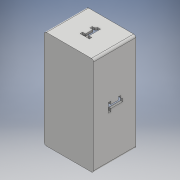
# Autodesk Inventor part: Контейнер 1
Saved by Autodesk Inventor 2018 (Build 220112000, 112)
## iProperties
Created: 2023-02-08
Part Number: Контейнер 1
Material: Типовые
Document SubType Name: Modeling
Designer: exper
Density: 1 g/cm^3
Appearance: По умолчанию
Author: exper
Autodesk Inventor part; units mm, degrees
ref_plane "YZ Plane" through (0, 0, 0) normal (1, 0, 0) x (0, 1, 0)
ref_plane "XZ Plane" through (0, 0, 0) normal (0, 1, 0) x (-1, 0, 0)
ref_plane "XY Plane" through (0, 0, 0) normal (0, 0, 1) x (1, 0, 0)
sketch "Эскиз1" plane through (0, 0, 0) normal (0, 1, 0) x (-1, 0, 0)
  line L0 (0, 0) -> (-70, 0)
  line L1 (-70, 0) -> (-70, -140)
  line L2 (-70, -140) -> (0, -140)
  line L3 (0, -140) -> (0, 0)
  dimension "d0" = 70
  dimension "d1" = 140
  constraints: 8 end point, 2 parallel, 1 horizontal, 1 perpendicular
  measures "d0" distance of L2.end L1.end
  measures "d1" distance of L1.end L0.end
extrude "Выдавливание1" add sketch "Эскиз1" along normal blind 60
shell "Оболочка1" thickness 3 removed faces 1 at (46.6667, 60, -93.3333)
sketch "Эскиз2" plane through (70, 0, 0) normal (1, 0, 0) x (0, 0, -1)
  line L0 (0, 60) -> (140, 60) projected
  line L1 (60.8364, 41.1842) -> (78.3566, 41.1842) construction
  line L2 (78.3566, 41.1842) -> (78.3566, 21.1356) construction
  line L3 (78.3566, 21.1356) -> (60.8364, 21.1356) construction
  line L4 (60.8364, 21.1356) -> (60.8364, 41.1842) construction
  line L5 (76.6711, 21.1356) -> (63.462, 21.1356)
  line L6 (63.462, 21.1356) -> (63.462, 24.6202)
  line L7 (63.462, 24.6202) -> (67.6759, 24.6202)
  line L8 (67.6759, 24.6202) -> (67.6759, 35.2037)
  line L9 (67.6759, 35.2037) -> (63.462, 35.2037)
  line L10 (63.462, 35.2037) -> (63.462, 38.4614)
  spline S0 degree 2 poles (63.462, 38.4614) (64.3858, 38.4614) (66.2172, 38.7045) (66.7683, 38.9638) knots 0 0 0 1 2 2 2
  spline S1 degree 2 poles (66.7683, 38.9638) (67.4004, 39.288) (68.1135, 40.3739) (68.1784, 41.1842) knots 0 0 0 1 2 2 2
  line L11 (68.1784, 41.1842) -> (72.5544, 41.1842)
  line L12 (72.5544, 41.1842) -> (72.5544, 24.6202)
  line L13 (72.5544, 24.6202) -> (76.6711, 24.6202)
  line L14 (76.6711, 24.6202) -> (76.6711, 21.1356)
  point P0 (0, 0)
  point P1 (70, 30.2829)
  constraints: 2 other
extrude "Выдавливание2" cut sketch "Эскиз2" against normal blind 12
sketch "Эскиз3" plane through (0, 0, 0) normal (0, 0, 1) x (1, 0, 0)
  line L0 (0, 60) -> (70, 60) projected
  line L1 (25.7932, 42.4372) -> (43.3135, 42.4372) construction
  line L2 (43.3135, 42.4372) -> (43.3135, 22.3886) construction
  line L3 (43.3135, 22.3886) -> (25.7932, 22.3886) construction
  line L4 (25.7932, 22.3886) -> (25.7932, 42.4372) construction
  line L5 (41.6279, 22.3886) -> (28.4189, 22.3886)
  line L6 (28.4189, 22.3886) -> (28.4189, 25.8732)
  line L7 (28.4189, 25.8732) -> (32.6328, 25.8732)
  line L8 (32.6328, 25.8732) -> (32.6328, 36.4566)
  line L9 (32.6328, 36.4566) -> (28.4189, 36.4566)
  line L10 (28.4189, 36.4566) -> (28.4189, 39.7143)
  spline S0 degree 2 poles (28.4189, 39.7143) (29.3427, 39.7143) (31.1741, 39.9575) (31.7252, 40.2168) knots 0 0 0 1 2 2 2
  spline S1 degree 2 poles (31.7252, 40.2168) (32.3573, 40.5409) (33.0704, 41.6268) (33.1352, 42.4372) knots 0 0 0 1 2 2 2
  line L11 (33.1352, 42.4372) -> (37.5112, 42.4372)
  line L12 (37.5112, 42.4372) -> (37.5112, 25.8732)
  line L13 (37.5112, 25.8732) -> (41.6279, 25.8732)
  line L14 (41.6279, 25.8732) -> (41.6279, 22.3886)
  point P0 (0, 0)
  point P1 (35, 31.2439)
  constraints: 2 other
extrude "Выдавливание3" cut sketch "Эскиз3" against normal blind 12
fillet "Сопряжение1" radius 3 4 edges at (3, 31.5, -3) (67, 31.5, -3) (3, 31.5, -137) (67, 31.5, -137)
fillet "Сопряжение2" radius 3 4 edges at (0, 30, -140) (0, 30, 0) (70, 30, -140) (70, 30, 0)
